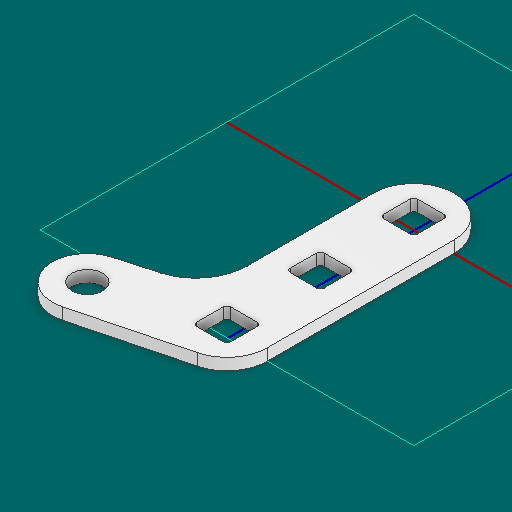
# Autodesk Inventor part: bent_gusset_improved
Saved by Autodesk Inventor 2025 (Build 290162000, 162)
## iProperties
Created: 2024-08-16
Part Number: bent_gusset_improved
Material: Acetal Resin, White
Document SubType Name: Modeling
Designer: averey
Density: 1.425 g/cm^3
Appearance: Smooth - White
d6: 0.182 in
d7: 0.182 in
d8: 0.020 in
d9: 0.500 in
d10: 0.500 in
d12: 0.675 in
Author: averey
Autodesk Inventor part; units mm, degrees
ref_plane "YZ Plane" through (0, 0, 0) normal (1, 0, 0) x (0, 1, 0)
ref_plane "XZ Plane" through (0, 0, 0) normal (0, 1, 0) x (-1, 0, 0)
ref_plane "XY Plane" through (0, 0, 0) normal (0, 0, 1) x (1, 0, 0)
sketch "hole" plane through (0, 0, 0) normal (0, 0, 1) x (1, 0, 0)
  line L0 (16.5616, -7.6441) -> (20.1684, -7.6441)
  line L1 (20.6764, -8.1521) -> (20.6764, -11.7589)
  line L2 (20.1684, -12.2669) -> (16.5616, -12.2669)
  line L3 (16.0536, -11.7589) -> (16.0536, -8.1521)
  line L4 (16.0536, -7.6441) -> (20.6764, -12.2669) construction
  line L5 (20.6764, -7.6441) -> (16.0536, -12.2669) construction
  arc A0 (20.6764, -8.1521) -> (20.1684, -7.6441) centre (20.1684, -8.1521) ccw
  arc A1 (20.1684, -12.2669) -> (20.6764, -11.7589) centre (20.1684, -11.7589) ccw
  arc A2 (16.0536, -11.7589) -> (16.5616, -12.2669) centre (16.5616, -11.7589) ccw
  arc A3 (16.5616, -7.6441) -> (16.0536, -8.1521) centre (16.5616, -8.1521) ccw
  point P0 (18.365, -9.9555)
  dimension "d6" = 4.6228
  dimension "d7" = 4.6228
  dimension "d8" = 0.508
  measures "d6" distance of L4.end L5.end
  measures "d7" distance of L5.start L4.end
  measures "d8" radius of A0
sketch "main" plane through (0, 0, 0) normal (0, 0, 1) x (1, 0, 0)
  arc A0 (12.865, -9.9555) -> (23.865, -9.9555) centre (18.365, -9.9555) ccw
  line L0 (12.865, 15.4445) -> (12.865, -9.9555)
  line L1 (23.865, -9.9555) -> (23.865, 7.1895)
  circle A1 centre (32.8381, 19.9475) radius 2.0955
  arc A2 (34.1305, 15.3637) -> (31.6462, 24.5584) centre (32.8381, 19.9475) ccw
  arc A3 (16.9885, 20.7695) -> (12.865, 15.4445) centre (18.365, 15.4445) ccw
  line L2 (16.9885, 20.7695) -> (31.6462, 24.5584)
  line L3 (34.1305, 15.3637) -> (28.9468, 13.9022)
  arc A4 (28.9468, 13.9022) -> (23.865, 7.1895) centre (30.8394, 7.1895) ccw
  line L4 (16.5616, -7.6441) -> (20.1684, -7.6441)
  line L5 (20.6764, -8.1521) -> (20.6764, -11.7589)
  line L6 (20.1684, -12.2669) -> (16.5616, -12.2669)
  line L7 (16.0536, -11.7589) -> (16.0536, -8.1521)
  line L8 (16.0536, -7.6441) -> (20.6764, -12.2669) construction
  line L9 (20.6764, -7.6441) -> (16.0536, -12.2669) construction
  arc A5 (20.6764, -8.1521) -> (20.1684, -7.6441) centre (20.1684, -8.1521) ccw
  arc A6 (20.1684, -12.2669) -> (20.6764, -11.7589) centre (20.1684, -11.7589) ccw
  arc A7 (16.0536, -11.7589) -> (16.5616, -12.2669) centre (16.5616, -11.7589) ccw
  arc A8 (16.5616, -7.6441) -> (16.0536, -8.1521) centre (16.5616, -8.1521) ccw
  line L10 (16.5616, 5.0559) -> (20.1684, 5.0559)
  line L11 (20.6764, 4.5479) -> (20.6764, 0.9411)
  line L12 (20.1684, 0.4331) -> (16.5616, 0.4331)
  line L13 (16.0536, 0.9411) -> (16.0536, 4.5479)
  line L14 (16.0536, 5.0559) -> (20.6764, 0.4331) construction
  line L15 (20.6764, 5.0559) -> (16.0536, 0.4331) construction
  arc A9 (20.6764, 4.5479) -> (20.1684, 5.0559) centre (20.1684, 4.5479) ccw
  arc A10 (20.1684, 0.4331) -> (20.6764, 0.9411) centre (20.1684, 0.9411) ccw
  arc A11 (16.0536, 0.9411) -> (16.5616, 0.4331) centre (16.5616, 0.9411) ccw
  arc A12 (16.5616, 5.0559) -> (16.0536, 4.5479) centre (16.5616, 4.5479) ccw
  line L16 (16.5616, 17.7559) -> (20.1684, 17.7559)
  line L17 (20.6764, 17.2479) -> (20.6764, 13.6411)
  line L18 (20.1684, 13.1331) -> (16.5616, 13.1331)
  line L19 (16.0536, 13.6411) -> (16.0536, 17.2479)
  line L20 (16.0536, 17.7559) -> (20.6764, 13.1331) construction
  line L21 (20.6764, 17.7559) -> (16.0536, 13.1331) construction
  arc A13 (20.6764, 17.2479) -> (20.1684, 17.7559) centre (20.1684, 17.2479) ccw
  arc A14 (20.1684, 13.1331) -> (20.6764, 13.6411) centre (20.1684, 13.6411) ccw
  arc A15 (16.0536, 13.6411) -> (16.5616, 13.1331) centre (16.5616, 13.6411) ccw
  arc A16 (16.5616, 17.7559) -> (16.0536, 17.2479) centre (16.5616, 17.2479) ccw
  point P0 (22.8879, 4.6952)
  dimension "d9" = 12.7
  dimension "d10" = 12.7
  dimension "d12" = 17.145
  measures "d12" distance of L1.start L1.end
sketch "Sketch1" plane through (0, 0, 0) normal (0, 1, 0) x (-1, 0, 0)
  arc A0 (-5.5, 0) -> (5.5, 0) centre (0, 0) ccw
  line L0 (-5.5, 25.4) -> (-5.5, 0)
  line L1 (5.5, 0) -> (5.5, 17.145)
  circle A1 centre (14.4731, 29.903) radius 2.0955
  arc A2 (15.7655, 25.3192) -> (13.2812, 34.5139) centre (14.4731, 29.903) ccw
  arc A3 (-1.3765, 30.725) -> (-5.5, 25.4) centre (0, 25.4) ccw
  line L2 (-1.3765, 30.725) -> (13.2812, 34.5139)
  line L3 (15.7655, 25.3192) -> (10.5818, 23.8577)
  arc A4 (10.5818, 23.8577) -> (5.5, 17.145) centre (12.4744, 17.145) ccw
  line L4 (-1.8034, 2.3114) -> (1.8034, 2.3114)
  line L5 (2.3114, 1.8034) -> (2.3114, -1.8034)
  line L6 (1.8034, -2.3114) -> (-1.8034, -2.3114)
  line L7 (-2.3114, -1.8034) -> (-2.3114, 1.8034)
  line L8 (-2.3114, 2.3114) -> (2.3114, -2.3114) construction
  line L9 (2.3114, 2.3114) -> (-2.3114, -2.3114) construction
  arc A5 (2.3114, 1.8034) -> (1.8034, 2.3114) centre (1.8034, 1.8034) ccw
  arc A6 (1.8034, -2.3114) -> (2.3114, -1.8034) centre (1.8034, -1.8034) ccw
  arc A7 (-2.3114, -1.8034) -> (-1.8034, -2.3114) centre (-1.8034, -1.8034) ccw
  arc A8 (-1.8034, 2.3114) -> (-2.3114, 1.8034) centre (-1.8034, 1.8034) ccw
  line L10 (-1.8034, 15.0114) -> (1.8034, 15.0114)
  line L11 (2.3114, 14.5034) -> (2.3114, 10.8966)
  line L12 (1.8034, 10.3886) -> (-1.8034, 10.3886)
  line L13 (-2.3114, 10.8966) -> (-2.3114, 14.5034)
  line L14 (-2.3114, 15.0114) -> (2.3114, 10.3886) construction
  line L15 (2.3114, 15.0114) -> (-2.3114, 10.3886) construction
  arc A9 (2.3114, 14.5034) -> (1.8034, 15.0114) centre (1.8034, 14.5034) ccw
  arc A10 (1.8034, 10.3886) -> (2.3114, 10.8966) centre (1.8034, 10.8966) ccw
  arc A11 (-2.3114, 10.8966) -> (-1.8034, 10.3886) centre (-1.8034, 10.8966) ccw
  arc A12 (-1.8034, 15.0114) -> (-2.3114, 14.5034) centre (-1.8034, 14.5034) ccw
  line L16 (-1.8034, 27.7114) -> (1.8034, 27.7114)
  line L17 (2.3114, 27.2034) -> (2.3114, 23.5966)
  line L18 (1.8034, 23.0886) -> (-1.8034, 23.0886)
  line L19 (-2.3114, 23.5966) -> (-2.3114, 27.2034)
  line L20 (-2.3114, 27.7114) -> (2.3114, 23.0886) construction
  line L21 (2.3114, 27.7114) -> (-2.3114, 23.0886) construction
  arc A13 (2.3114, 27.2034) -> (1.8034, 27.7114) centre (1.8034, 27.2034) ccw
  arc A14 (1.8034, 23.0886) -> (2.3114, 23.5966) centre (1.8034, 23.5966) ccw
  arc A15 (-2.3114, 23.5966) -> (-1.8034, 23.0886) centre (-1.8034, 23.5966) ccw
  arc A16 (-1.8034, 27.7114) -> (-2.3114, 27.2034) centre (-1.8034, 27.2034) ccw
  constraints: 1 other
extrude "Extrusion1" add sketch "Sketch1" along normal blind 1.5875
body "Solid1"
